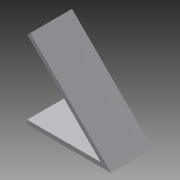
# Autodesk Inventor part: Reinforcer_Front
Saved by Autodesk Inventor 2013 (Build 170138000, 138)
## iProperties
Created: 2015-07-03
Part Number: Reinforcer_Front
Material: Aluminum 6061
Document SubType Name: Modeling
Designer: Kyle
Mass: 2.49079 g
Surface Area: 16.2442 cm^2
Volume: 0.919111 cm^3
Density: 2.71 g/cm^3
Author: Kyle
Autodesk Inventor part; units mm, degrees
ref_plane "YZ Plane" through (0, 0, 0) normal (1, 0, 0) x (0, 1, 0)
ref_plane "XZ Plane" through (0, 0, 0) normal (0, 1, 0) x (-1, 0, 0)
ref_plane "XY Plane" through (0, 0, 0) normal (0, 0, 1) x (1, 0, 0)
sketch "Sketch1" plane through (0, 0, 0) normal (0, 0, 1) x (1, 0, 0)
  line L0 (0, 0) -> (0, 25.4)
  line L1 (0, 25.4) -> (25.4, 0)
  line L2 (25.4, 0) -> (0, 0)
  dimension "d0" = 25.4
  dimension "d1" = 25.4
  constraints: 6 end point, 1 perpendicular, 1 vertical
  measures "d0" distance of L0.start L0.end
  measures "d1" distance of L1.end L0.start
extrude "Extrusion1" add sketch "Sketch1" along normal blind 12.7
sketch "Sketch2" plane through (0, 0, 12.7) normal (0, 0, 1) x (1, 0, 0)
  line L0 (0, 25.4) -> (0, 0) projected
  line L1 (0, 0) -> (25.4, 0) projected
  line L2 (25.4, 0) -> (0, 25.4) projected
  line L3 (1.27, 1.27) -> (22.3339, 1.27)
  line L4 (22.3339, 1.27) -> (1.27, 22.3339)
  line L5 (1.27, 1.27) -> (0, 1.27)
  line L6 (1.27, 22.3339) -> (0, 23.6039)
  line L7 (0, 23.6039) -> (0.898, 24.502)
  line L8 (0, 1.27) -> (0, 23.6039)
  line L9 (0, 23.6039) -> (0, 25.4)
  line L10 (0, 25.4) -> (0.898, 24.502)
  dimension "d4" = 1.27
  constraints: 16 end point, 4 collinear, 3 point on line, 2 perpendicular, 1 other
  measures "d4" distance between parallel lines of L1 L3
extrude "Extrusion2" cut sketch "Sketch2" against normal blind 25.4 contours L2 L7 L0 | L6 L4 L3 L5 L0
body "Solid1"
